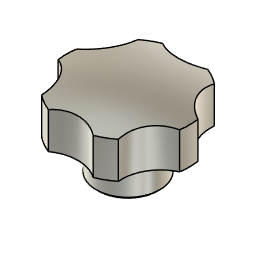
35 (Autodesk Fusion 360 design; units mm, degrees)
Autodesk Fusion 360 part; units mm, degrees
sketch "草图1" plane through (0, 0, 0) normal (0, 1, 0) x (1, 0, 0)
  line L0 (0, -75) -> (0, 75) construction
  line L1 (0, 20) -> (13, 20)
  line L2 (14, 19) -> (14, 5.8348)
  line L3 (16, 3.8348) -> (27, 3.8348)
  line L4 (27, 3.8348) -> (27, -12.1652)
  line L5 (0, 20) -> (0, -15)
  arc A0 (0, -15) -> (27, -12.1652) centre (0, 115) ccw
  arc A1 (14, 5.8348) -> (16, 3.8348) centre (16, 5.8348) ccw
  line L6 (13, 20) -> (14, 19)
  point P0 (14, 20)
  dimension "d1" = 20
  dimension "d2" = 14
  dimension "d3" = 16
  dimension "d4" = 35
  dimension "d5" = 130
  dimension "d6" = 27
  dimension "d7" = 2
  dimension "d8" = 1
  dimension "d9" = 45
  constraint vertical L0
  constraint coincident L0 L1.start
  constraint perpendicular L0 L1
  constraint perpendicular L1 L2
  constraint perpendicular L0 L3
  constraint perpendicular L3 L4
  constraint coincident L0 L5.end
  constraint collinear L0.start L0.end A0.centre
  constraint tangent L2 A1
  constraint tangent L3 A1
  constraint coincident P0 L1
  constraint coincident P0 L2
  measures "d1" distance of origin L1.start
  measures "d2" distance of L1.start P0
  measures "d3" distance of L3.end L4.end
  measures "d4" distance of L1.start L5.end
  measures "d5" radius of A0
  measures "d6" horizontal distance of L1.start L3.end
  measures "d7" radius of A1
  measures "d8" distance of P0 L1.end
  measures "d9" angle of L1 L6
revolve "旋转1" add sketch "草图1" angle 360 about axis through (0, 0, 75) along (0, 0, -1)
sketch "草图2" plane through (0, 0, 0) normal (0, 0, 1) x (1, 0, 0)
  circle A0 centre (0, 0) radius 27
  circle A1 centre (0, 0) radius 22 construction
  arc A2 (-9.8452, 25.141) -> (9.8452, 25.141) centre (0, 39) ccw
  line L0 (0, 40) -> (0, -45) construction
  arc A3 (-26.6954, 4.0443) -> (-16.8501, 21.0967) centre (-33.775, 19.5) ccw
  arc A4 (-16.8501, -21.0967) -> (-26.6954, -4.0443) centre (-33.775, -19.5) ccw
  arc A5 (9.8452, -25.141) -> (-9.8452, -25.141) centre (0, -39) ccw
  arc A6 (26.6954, -4.0443) -> (16.8501, -21.0967) centre (33.775, -19.5) ccw
  arc A7 (16.8501, 21.0967) -> (26.6954, 4.0443) centre (33.775, 19.5) ccw
  dimension "d11" = 54
  dimension "d12" = 44
  dimension "d13" = 17
  dimension "d15" = 360
  constraint coincident A0.centre A1.centre
  constraint concentric A0 A1
  constraint tangent A1 A2
  constraint coincident A0 A2.end
  constraint coincident A0 A2.start
  constraint vertical L0
  constraint symmetric A2.start A2.end L0
  measures "d11" diameter of A0
  measures "d12" diameter of A1
  measures "d13" radius of A2
extrude "拉伸1" cut sketch "草图2" along normal through all and the other way through all contours A0 A2 A3 A4 A5 A6 A7 keep common part
hole "孔1" at (0, 0, -20) direction (0, 0, 1) diameter 10 depth 20 tip angle 118
